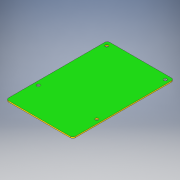
# Autodesk Inventor part: RasPI
Saved by Autodesk Inventor 2019 (Build 230136000, 136)
## iProperties
Created: 2019-02-12
Part Number: RasPI
Material: Generic
Document SubType Name: Modeling
Designer: izsoandras
Density: 1 g/cm^3
Appearance: Default
Author: izsoandras
Autodesk Inventor part; units mm, degrees
ref_plane "YZ Plane" through (0, 0, 0) normal (1, 0, 0) x (0, 1, 0)
ref_plane "XZ Plane" through (0, 0, 0) normal (0, 1, 0) x (-1, 0, 0)
ref_plane "XY Plane" through (0, 0, 0) normal (0, 0, 1) x (1, 0, 0)
sketch "Sketch1" plane through (0, 0, 0) normal (0, 1, 0) x (-1, 0, 0)
  line L0 (20.1466, 45.9072) -> (-31.8534, 45.9072)
  line L1 (-33.8534, 43.9072) -> (-33.8534, -37.0928)
  line L2 (-31.8534, -39.0928) -> (20.1466, -39.0928)
  line L3 (22.1466, -37.0928) -> (22.1466, 43.9072)
  arc A0 (22.1466, 43.9072) -> (20.1466, 45.9072) centre (20.1466, 43.9072) ccw
  arc A1 (20.1466, -39.0928) -> (22.1466, -37.0928) centre (20.1466, -37.0928) ccw
  arc A2 (-33.8534, -37.0928) -> (-31.8534, -39.0928) centre (-31.8534, -37.0928) ccw
  arc A3 (-31.8534, 45.9072) -> (-33.8534, 43.9072) centre (-31.8534, 43.9072) ccw
  point P0 (0, 0)
  point P1 (22.1466, 45.9072)
  point P2 (-33.8534, -39.0928)
  point P3 (-33.8534, 45.9072)
  point P4 (22.1466, -39.0928)
  dimension "d0" = 85
  dimension "d1" = 56
  dimension "d4" = 2
  constraints: 8 end point, 8 point on circle, 8 point on line, 8 tangent, 4 centre point, 3 equal radius, 2 parallel, 1 horizontal, 1 perpendicular
  measures "d0" distance of point (22.147, -39.093) point (22.147, 45.907)
  measures "d1" distance of point (22.147, 45.907) point (-33.853, 45.907)
  measures "d4" radius of A0
extrude "Extrusion1" add sketch "Sketch1" along normal blind 1
sketch "Sketch2" plane through (0, 1, 0) normal (0, 1, 0) x (1, 0, 0)
  circle A0 centre (-18.6966, 35.2428) radius 1.25
  line L0 (-22.1466, 37.0928) -> (-22.1466, -43.9072) projected
  line L1 (31.8534, 39.0928) -> (-20.1466, 39.0928) projected
  circle A1 centre (30.4034, 35.2428) radius 1.25
  circle A2 centre (-18.6966, -22.2572) radius 1.25
  circle A3 centre (30.4034, -22.2572) radius 1.25
  line L2 (33.8534, -43.9072) -> (33.8534, 37.0928) projected
  point P0 (0, 0)
  dimension "d5" = 2.5
  dimension "d6" = 3.45
  dimension "d7" = 3.85
  dimension "d8" = 2.5
  dimension "d9" = 3.85
  dimension "d10" = 3.45
  dimension "d11" = 2.5
  dimension "d12" = 3.45
  dimension "d13" = 57.5
  dimension "d14" = 57.5
  dimension "d15" = 2.5
  dimension "d16" = 3.45
  constraints: 4 centre point
  measures "d5" diameter of A0
  measures "d6" distance from line of L0 A0.centre
  measures "d7" distance from line of L1 A0.centre
  measures "d8" diameter of A1
  measures "d9" distance from line of L1 A1.centre
  measures "d10" distance from line of L2 A1.centre
  measures "d11" diameter of A2
  measures "d12" distance from line of L0 A2.centre
  measures "d13" distance of A0.centre A2.centre
  measures "d14" distance of A1.centre A3.centre
  measures "d15" diameter of A3
  measures "d16" distance from line of L2 A3.centre
extrude "Extrusion2" cut sketch "Sketch2" against normal up to next
equation "\"d8\" = d5"
equation "\"d9\" = d7"
equation "\"d10\" = d6"
equation "\"d11\" = d5"
equation "\"d12\" = d6"
equation "\"d14\" = d13"
equation "\"d15\" = d5"
equation "\"d16\" = d6"
body "Solid1"
